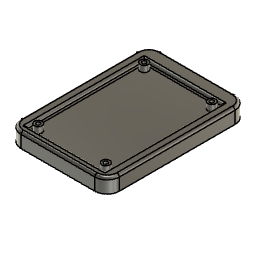
PCB Holder For Test Stand (Autodesk Fusion 360 design; units mm, degrees)
Autodesk Fusion 360 part; units mm, degrees
note: some values were not read from the file. Set by a fixed rule: which sketch regions a step uses.
sketch "Sketch1" plane through (0, 0, 0) normal (0, 0, 1) x (1, 0, 0)
  line L0 (-25.4, 38.1) -> (25.4, 38.1)
  line L1 (25.4, 38.1) -> (25.4, -34.29)
  line L2 (25.4, -34.29) -> (-25.4, -34.29)
  line L3 (-25.4, -34.29) -> (-25.4, 38.1)
  dimension "d1" = 50.8
  dimension "d2" = 72.39
  constraint horizontal L0
  constraint vertical L1
  constraint horizontal L2
  constraint vertical L3
  measures "d1" distance of L0.start L0.end
  measures "d2" distance of L0.start L2.end
extrude "Extrude1" add sketch "Sketch1" along normal blind 7.62
sketch "Sketch2" plane through (0, 0, 0) normal (0, 0, -1) x (1, 0, 0)
  line L0 (25.4, 34.29) -> (-25.4, 34.29)
  line L1 (-25.4, 34.29) -> (-25.4, -38.1)
  line L2 (-25.4, -38.1) -> (25.4, -38.1)
  line L3 (25.4, -38.1) -> (25.4, 34.29)
  circle A0 centre (0, 0) radius 3.937
  dimension "d5" = 7.874
  constraint coincident A0.centre origin
  measures "d5" diameter of A0
extrude "Extrude2" add sketch "Sketch2" along normal blind 6.985 contours A0
sketch "Sketch3" plane through (0, 0, 7.62) normal (0, 0, 1) x (-1, 0, 0)
  line L0 (25.4, 34.29) -> (-25.4, 34.29)
  line L1 (-25.4, 34.29) -> (-25.4, -38.1)
  line L2 (-25.4, -38.1) -> (25.4, -38.1)
  line L3 (25.4, -38.1) -> (25.4, 34.29)
  line L4 (0, 0) -> (-19.939, 0)
  line L5 (-19.939, 0) -> (-19.939, 29.972)
  line L6 (-19.939, 29.972) -> (19.939, 29.972)
  line L7 (19.939, 29.972) -> (19.939, -30.226)
  line L8 (19.939, -30.226) -> (-19.939, -30.226)
  line L9 (-19.939, -30.226) -> (-19.939, 29.972)
  dimension "d8" = 19.939
  dimension "d9" = 29.972
  dimension "d10" = 39.878
  dimension "d11" = 60.198
  constraint coincident L4.start origin
  constraint perpendicular L1 L4
  constraint perpendicular L4 L5
  constraint horizontal L6
  constraint vertical L7
  constraint horizontal L8
  constraint vertical L9
  measures "d8" distance of L4.start L4.end
  measures "d9" distance of L4.end L5.end
  measures "d10" distance of L5.end L6.end
  measures "d11" distance of L5.end L8.end
extrude "Extrude3" cut sketch "Sketch3" against normal blind 2.54 contours L5 L6 L7 L8 L9
fillet "Fillet1" radius 1.27 4 edges at (19.939, 0.127, 7.62) (0, -29.972, 7.62) (-19.939, 0.127, 7.62) (0, 30.226, 7.62)
fillet "Fillet2" radius 6.35 4 edges at (-25.4, 38.1, 3.81) (-25.4, -34.29, 3.81) (25.4, -34.29, 3.81) (25.4, 38.1, 3.81)
sketch "Sketch4" plane through (0, 0, 5.08) normal (0, 0, 1) x (-1, 0, 0)
  line L0 (-19.939, -30.226) -> (19.939, -30.226)
  line L1 (19.939, -30.226) -> (19.939, 29.972)
  line L2 (19.939, 29.972) -> (-19.939, 29.972)
  line L3 (-19.939, 29.972) -> (-19.939, -30.226)
  line L4 (19.939, -30.226) -> (17.5578, -30.226)
  line L5 (17.5578, -30.226) -> (17.5578, -27.8448)
  line L6 (17.5578, -27.8448) -> (-17.3673, -27.8448)
  line L7 (-17.3673, -27.8448) -> (-17.3673, 26.924)
  line L8 (17.5578, -27.8448) -> (-17.3673, -27.8448)
  line L9 (-17.3673, -27.8448) -> (-17.3673, 26.924)
  line L10 (-17.3673, 26.924) -> (17.5578, 26.924)
  line L11 (17.5578, 26.924) -> (17.5578, -27.8448)
  circle A0 centre (17.5578, 26.924) radius 2.032
  circle A1 centre (17.5578, -27.8448) radius 2.032
  circle A2 centre (-17.3673, -27.8448) radius 2.032
  circle A3 centre (-17.3673, 26.924) radius 2.032
  dimension "d18" = 2.3813
  dimension "d19" = 2.3813
  dimension "d20" = 34.925
  dimension "d21" = 54.7687
  dimension "d22" = 4.064
  dimension "d23" = 4.064
  dimension "d24" = 4.064
  dimension "d25" = 4.064
  constraint coincident L0.end L1.start
  constraint perpendicular L1 L4
  constraint perpendicular L4 L5
  constraint perpendicular L5 L6
  constraint perpendicular L6 L7
  constraint horizontal L8
  constraint vertical L9
  constraint horizontal L10
  constraint vertical L11
  constraint coincident L10.end L11.start
  constraint coincident L5.end L6.start
  constraint coincident L6.end L7.start
  constraint coincident L7.end L9.end
  measures "d18" distance of L0.end L4.end
  measures "d19" distance of L4.end L5.end
  measures "d20" distance of L5.end L6.end
  measures "d21" distance of L6.end L7.end
  measures "d22" diameter of A0
  measures "d23" diameter of A1
  measures "d24" diameter of A2
  measures "d25" diameter of A3
extrude "Extrude4" add sketch "Sketch4" along normal blind 3.175 contours L5 L6 L8 A1 | L5 L11 A1 | L6 L8 L11 A1 | L6 L7 L8 L9 A2 | L6 L7 L8 L9 A2 | L10 L11 A0 | L10 L11 A0 | L7 L9 L10 A3 | L7 L9 L10 A3
sketch "Sketch5" plane through (0, 0, 8.255) normal (0, 0, 1) x (-1, 0, 0)
  circle A0 centre (17.5578, -27.8448) radius 2.032
  circle A1 centre (17.5578, -27.8448) radius 1.016
  dimension "d28" = 2.032
  constraint concentric A0 A1
  measures "d28" diameter of A1
sketch "Sketch6" plane through (0, 0, 8.255) normal (0, 0, 1) x (-1, 0, 0)
  circle A0 centre (-17.3673, -27.8448) radius 2.032
  circle A1 centre (-17.3673, -27.8448) radius 1.016
  dimension "d29" = 2.032
  constraint concentric A0 A1
  measures "d29" diameter of A1
sketch "Sketch7" plane through (0, 0, 8.255) normal (0, 0, 1) x (-1, 0, 0)
  circle A0 centre (17.5578, 26.924) radius 2.032
  circle A1 centre (17.5578, 26.924) radius 1.016
  dimension "d30" = 2.032
  constraint concentric A0 A1
  measures "d30" diameter of A1
sketch "Sketch8" plane through (0, 0, 8.255) normal (0, 0, 1) x (-1, 0, 0)
  circle A0 centre (-17.3673, 26.924) radius 2.032
  circle A1 centre (-17.3673, 26.924) radius 1.016
  dimension "d31" = 2.032
  constraint concentric A0 A1
  measures "d31" diameter of A1
extrude "Extrude5" cut sketch "Sketch5" sketch "Sketch7" sketch "Sketch6" sketch "Sketch8" against normal blind 5.08 contours A1 of sketch 2 contours A1 of sketch 3 contours A1 of sketch 4 contours A1
fillet "Fillet3" radius 1.27 8 edges at (23.5401, -32.4301, 7.62) (25.4, 1.905, 7.62) (23.5401, 36.2401, 7.62) (0, 38.1, 7.62) (-23.5401, 36.2401, 7.62) (-25.4, 1.905, 7.62) (-23.5401, -32.4301, 7.62) (0, -34.29, 7.62)
equation "d8 = ( 1.57 / 2 ) * 1 in"
equation "d9 = ( 2.36 / 2 ) * 1 in"
equation "d18 = ( 3 / 32 ) * 1 in"
equation "d19 = ( 3 / 32 ) * 1 in"
equation "d26 = ( 1 / 8 ) * 1 in"
